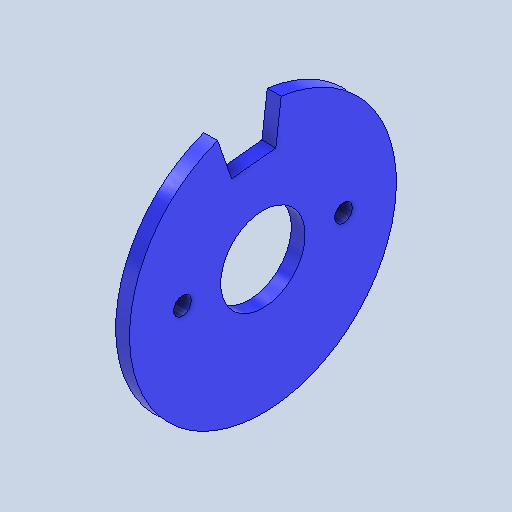
# Autodesk Inventor part: belt_liner_v2_3DP_P-3-F
Saved by Autodesk Inventor 2025.2 (Build 292293000, 293)
## iProperties
Created: 2025-01-13
Part Number: belt_liner_v2_3DP_P-3-F
Material: ABS プラスチック
Document SubType Name: Modeling
Designer: haruy
Density: 1.06 g/cm^3
Appearance: 青 - 壁塗料 - 光沢
Author: haruy
Autodesk Inventor part; units mm, degrees
ref_plane "YZ Plane" through (0, 0, 0) normal (1, 0, 0) x (0, 1, 0)
ref_plane "XZ Plane" through (0, 0, 0) normal (0, 1, 0) x (-1, 0, 0)
ref_plane "XY Plane" through (0, 0, 0) normal (0, 0, 1) x (1, 0, 0)
sketch "スケッチ2" plane through (0, 0, 0) normal (1, 0, 0) x (0, 1, 0)
  line L0 (20.1406, 10.7459) -> (27.3588, 13.2667)
  arc A0 (27.3588, 13.2667) -> (28.5614, 1.8249) centre (4.7873, 5.1102) ccw
  line L1 (28.5614, 1.8249) -> (20.9768, 2.7898)
  line L2 (20.9768, 2.7898) -> (20.1406, 10.7459)
  circle A1 centre (4.7873, 19.6102) radius 1.6
  circle A2 centre (4.7873, -9.3898) radius 1.6
  circle A3 centre (4.7873, 5.1102) radius 7.6
  point P0 (0, 0)
  constraints: 6 end point, 4 centre point, 2 point on circle
extrude "押し出し2" add sketch "スケッチ2" along normal blind 2.5
